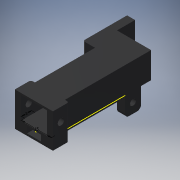
# Autodesk Inventor part: motoruchyt
Saved by Autodesk Inventor 2016 (Build 200138000, 138)
## iProperties
Created: 2015-05-23
Part Number: motoruchyt
Material: ABS Plastic
Document SubType Name: Modeling
Designer: Jufo
Density: 1 g/cm^3
Appearance: Smooth - White
Author: Jufo
Autodesk Inventor part; units mm, degrees
ref_plane "YZ Plane" through (0, 0, 0) normal (1, 0, 0) x (0, 1, 0)
ref_plane "XZ Plane" through (0, 0, 0) normal (0, 1, 0) x (-1, 0, 0)
ref_plane "XY Plane" through (0, 0, 0) normal (0, 0, 1) x (1, 0, 0)
sketch "Sketch1" plane through (0, 0, 0) normal (0, 1, 0) x (-1, 0, 0)
  line L0 (0, 6.5) -> (-5.5, 6.5)
  line L1 (-5.5, 6.5) -> (-5.5, -4.5)
  line L2 (-5.5, -4.5) -> (7.5, -4.5)
  line L3 (7.5, -4.5) -> (7.5, 6.5)
  line L4 (7.5, 6.5) -> (0, 6.5)
  line L5 (8.5, 7.5) -> (8.5, -5.5)
  line L6 (8.5, -5.5) -> (-6.5, -5.5)
  line L7 (-6.5, -5.5) -> (-6.5, 7.5)
  line L8 (-6.5, 7.5) -> (8.5, 7.5)
  point P0 (0, 0)
  dimension "d2" = 11
  dimension "d3" = 13
  dimension "d6" = 13
  dimension "d7" = 15
  dimension "d47" = 1
  dimension "d48" = 1
  constraints: 18 end point, 5 perpendicular, 1 collinear, 1 parallel
  measures "d2" distance of L0.end L1.end
  measures "d3" distance of L1.end L2.end
  measures "d6" distance of L5.start L5.end
  measures "d7" distance of L5.end L6.end
  measures "d47" distance between parallel lines of L8 L0
  measures "d48" distance between parallel lines of L1 L7
extrude "Extrusion1" add sketch "Sketch1" along normal blind 50
sketch "Sketch2" plane through (0, 50, 0) normal (0, 1, 0) x (1, 0, 0)
  line L0 (-8.5, 5.5) -> (-8.5, -7.5) projected
  line L1 (-8.5, -7.5) -> (6.5, -7.5) projected
  line L2 (6.5, -7.5) -> (6.5, 5.5) projected
  line L3 (6.5, 5.5) -> (-8.5, 5.5) projected
  circle A0 centre (0, 0) radius 2.5
  circle A1 centre (-4, 0) radius 0.75
  circle A2 centre (4, 0) radius 0.75
  dimension "d10" = 5
  dimension "d14" = 1.5
  constraints: 3 centre point, 1 coincident
  measures "d10" diameter of A0
  measures "d14" diameter of A1
extrude "Extrusion2" add sketch "Sketch2" along normal blind 1
sketch "Sketch3" plane through (6.5, 0, 7.5) normal (1, 0, 0) x (0, 0, -1)
  line L0 (0, 51) -> (13, 51) projected
  line L1 (0, 0) -> (0, 51) projected
  line L2 (6.5, 51) -> (6.5, 4)
  circle A0 centre (6.5, 4) radius 1.6
  point P0 (7.5, 0)
  dimension "d17" = 47
  dimension "d18" = 3.2
  constraints: 2 end point, 1 centre point, 1 coincident, 1 midpoint, 1 parallel
  measures "d17" distance of L2.start L2.end
  measures "d18" diameter of A0
extrude "Extrusion3" cut sketch "Sketch3" against normal blind 50
sketch "Sketch7" plane through (6.5, 0, -5.5) normal (0, 0, -1) x (-1, 0, 0)
  line L0 (0, 43) -> (0, 46)
  line L1 (0, 46) -> (4, 46)
  line L2 (4, 46) -> (4, 38)
  line L3 (4, 38) -> (0, 38)
  line L4 (0, 38) -> (0, 43)
  line L5 (11, 46) -> (11, 38)
  line L6 (11, 38) -> (15, 38)
  line L7 (15, 38) -> (15, 46)
  line L8 (15, 46) -> (11, 46)
  line L9 (0, 0) -> (0, 51) projected
  line L10 (0, 51) -> (15, 51) projected
  point P0 (6.5, 0)
  dimension "d33" = 3
  dimension "d34" = 8
  dimension "d35" = 7
  dimension "d36" = 4
  dimension "d37" = 4
  dimension "d38" = 8
  dimension "d55" = 0
  dimension "d92" = 7
  dimension "d93" = 5
  constraints: 18 end point, 4 perpendicular, 1 collinear, 1 parallel, 1 point on line
  measures "d33" distance of L0.start L0.end
  measures "d34" distance of L1.end L2.end
  measures "d35" distance of L1.end L5.start
  measures "d36" distance of L0.end L1.end
  measures "d37" distance of L5.end L6.end
  measures "d38" distance of L5.start L5.end
  measures "d55" distance between parallel lines of L9 L4
  measures "d92" distance of L5.end L2.end
  measures "d93" distance between parallel lines of L10 L1
extrude "Extrusion7" add sketch "Sketch7" along normal blind 10
sketch "Sketch9" plane through (0, 51, 0) normal (0, 1, 0) x (1, 0, 0)
  circle A0 centre (0, 0) radius 2.5 projected
  circle A1 centre (4, 0) radius 0.75 projected
  circle A2 centre (-4, 0) radius 0.75 projected
  circle A3 centre (-4, 0) radius 0.75
  circle A4 centre (4, 0) radius 0.75
  circle A5 centre (0, 0) radius 2.5
  constraints: 3 centre point, 3 coincident, 3 concentric
extrude "Extrusion9" add sketch "Sketch9" against normal blind 1
sketch "Sketch11" plane through (0, 51, 0) normal (0, 1, 0) x (1, 0, 0)
  line L0 (2.5, 5.5) -> (-4.5, 5.5) projected
  line L1 (6.5, 5.5) -> (-1, 5.5)
  line L2 (-1, 5.5) -> (-1, -1)
  circle A0 centre (-1, -1) radius 2.5
  point P0 (-17.5, 5.5)
  point P1 (0, 0)
  point P2 (-18.5, 5.5)
  point P3 (-8.5, 5.5)
  dimension "d51" = 7.5
  dimension "d52" = 5
  constraints: 4 end point, 1 centre point, 1 coincident, 1 midpoint, 1 perpendicular
  measures "d51" distance of L1.start L1.end
  measures "d52" diameter of A0
extrude "Extrusion10" cut sketch "Sketch11" against normal blind 1
sketch "Sketch12" plane through (6.5, 0, 7.5) normal (1, 0, 0) x (0, 0, -1)
  circle A0 centre (18.05, 42) radius 1.5
  line L0 (13, 38) -> (23, 38) projected
  line L1 (13, 46) -> (23, 46) projected
  point P0 (7.5, 0)
  dimension "d56" = 3
  dimension "d144" = 4
  dimension "d145" = 4
  constraints: 1 centre point
  measures "d56" diameter of A0
  measures "d144" distance from line of L0 A0.centre
  measures "d145" distance from line of A0.centre L1
extrude "Extrusion11" cut sketch "Sketch12" against normal blind 15
sketch "Sketch16" plane through (-8.5, 39, -13.5) normal (-1, 0, 0) x (0, 0, 1)
  line L0 (21, -39) -> (8, -39) projected
  circle A0 centre (14.5, -35) radius 1.6 projected
  line L1 (8, -39) -> (8, -1) projected
  line L2 (21, -39) -> (21, 12) projected
  line L3 (8, -31) -> (21, -31)
  dimension "d147" = 8
  constraints: 2 end point, 2 point on line, 1 perpendicular
  measures "d147" distance between parallel lines of L3 L0
extrude "Extrusion15" add sketch "Sketch16" along normal blind 2
sketch "Sketch17" plane through (6.5, 0, 7.5) normal (1, 0, 0) x (0, 0, -1)
  circle A0 centre (6.5, 4) radius 1.6 projected
  line L0 (0, 0) -> (0, 51) projected
  line L1 (13, 0) -> (0, 0) projected
  line L2 (13, 0) -> (13, 38) projected
  line L3 (13, 46) -> (23, 46) projected
  line L4 (6.5, 0) -> (6.5, 8)
  line L5 (0, 21) -> (13, 21)
  line L6 (0, 0) -> (0, 51) projected
  line L7 (0, 8) -> (13, 8)
  point P0 (7.5, 0)
  dimension "d78" = 8
  constraints: 6 end point, 4 point on line, 3 perpendicular, 1 midpoint
  measures "d78" distance of L4.start L4.end
fillet "Fillet11" radius 2 4 edges at (4.5, 46, -15.5) (4.5, 38, -15.5) (-6.5, 46, -15.5) (-6.5, 38, -15.5)
extrude "Extrusion18" add sketch "Sketch17" along normal blind 2 contours A0 L4 L7 L2 L1 | A0 L4 L1 L0 L7
sketch "Sketch21" plane through (-8.5, 8, 7.5) normal (-1, 0, 0) x (0, 0, 1)
  line L0 (-13, 52) -> (-13, 30)
  line L1 (0, 52) -> (0, 30)
  line L2 (0, 0) -> (0, 43) projected
  line L3 (-13, 38) -> (-13, 30) projected
  line L4 (-13, 30) -> (0, 30)
  line L5 (-13, 43) -> (0, 43) projected
  line L6 (-13, 52) -> (0, 52)
  constraints: 8 end point, 2 perpendicular, 1 horizontal, 1 point on line
extrude "Extrusion19" add sketch "Sketch21" along normal blind 6
sketch "Sketch31" plane through (0, 51, 0) normal (0, 1, 0) x (1, 0, 0)
  circle A0 centre (-1, -1) radius 2.5 projected
  line L0 (-1, -1) -> (3.45, -1)
  line L1 (5.5, -6.5) -> (5.5, 4.5) projected
  circle A1 centre (3.45, -1) radius 0.7
  line L2 (-1, -1) -> (-5.45, -1)
  circle A2 centre (-5.45, -1) radius 0.7
  point P0 (0, 0)
  dimension "d150" = 4.45
  dimension "d151" = 1.4
  dimension "d153" = 4.45
  dimension "d154" = 1.4
  dimension "d253" = 10.3
  constraints: 4 end point, 2 centre point, 2 coincident, 1 horizontal, 1 perpendicular
  measures "d150" distance of L0.start L0.end
  measures "d151" diameter of A1
  measures "d153" distance of L0.start L2.end
  measures "d154" diameter of A2
extrude "Extrusion28" cut sketch "Sketch31" against normal blind 2 contours A1 | A2
sketch "Sketch32" plane through (-14.5, 8, 7.5) normal (-1, 0, 0) x (0, 0, 1)
  line L0 (0, 30) -> (0, 52) projected
  line L1 (-13, 30) -> (0, 30) projected
  line L2 (-9.5, 50) -> (-3.5, 50)
  line L3 (-3.5, 50) -> (-3.5, 40)
  line L4 (-3.5, 40) -> (-9.5, 40)
  line L5 (-9.5, 40) -> (-9.5, 50)
  line L6 (-13, 52) -> (-13, 30) projected
  point P0 (-7.5, -8)
  dimension "d160" = 10
  dimension "d162" = 3.5
  dimension "d235" = 6
  dimension "d236" = 3.5
  constraints: 8 end point, 2 parallel, 1 horizontal, 1 perpendicular
  measures "d160" distance of L4.end L2.start
  measures "d162" distance between parallel lines of L0 L3
  measures "d235" distance of L2.start L2.end
  measures "d236" distance between parallel lines of L6 L5
extrude "Extrusion29" cut sketch "Sketch32" against normal blind 3
sketch "Sketch39" plane through (6.5, 46, -5.5) normal (0, 0, -1) x (-1, 0, 0)
  line L0 (4, 0) -> (4, -8) projected
  line L1 (-2, -46) -> (-2, -38) projected
  line L2 (-2, -46) -> (-2, -38)
  line L3 (0, -38) -> (-2, -38) projected
  line L4 (-2, -38) -> (0, -38)
  line L5 (0, -38) -> (0, -8)
  line L6 (0, -38) -> (0, -8) projected
  line L7 (0, -8) -> (4, -8)
  line L8 (15, -8) -> (11, -8) projected
  line L9 (11, -8) -> (15, -8)
  line L10 (15, -8) -> (15, -38)
  line L11 (15, -38) -> (17, -38) projected
  line L12 (15, -38) -> (17, -38)
  line L13 (17, -38) -> (17, -46) projected
  line L14 (17, -38) -> (17, -46)
  line L15 (17, -46) -> (-2, -46)
  line L16 (11, -8) -> (11, -46)
  line L17 (14, -46) -> (1, -46) projected
  line L18 (3, -8) -> (4, -8)
  line L19 (11, -8) -> (12, -8)
  line L20 (11, -8) -> (15, -8) projected
  line L21 (12, -8) -> (12, -46)
  line L22 (11, -46) -> (12, -46)
  line L23 (3, -8) -> (4, -8)
  line L24 (4, -8) -> (0, -8) projected
  line L25 (4, -8) -> (3, -8)
  line L26 (3, -8) -> (3, -46)
  line L27 (3, -46) -> (4, -46)
  line L28 (4, -46) -> (4, -8)
  line L29 (15, -38) -> (15, -8) projected
  line L30 (12, -8) -> (15, -8)
  line L31 (15, -8) -> (15, -13)
  line L32 (15, -13) -> (12, -13)
  line L33 (12, -13) -> (12, -8)
  line L34 (4, -8) -> (11, -8)
  line L35 (4, -9) -> (11, -9)
  line L36 (4, -9) -> (4, -12)
  line L37 (4, -9) -> (7, -9)
  arc A0 (7, -9) -> (4, -12) centre (7, -12) ccw
  line L38 (4, -12) -> (4, -46)
  line L39 (7, -9) -> (11, -9)
  line L40 (12, -38) -> (15, -38)
  line L41 (12, -39) -> (16, -39)
  line L42 (16, -39) -> (16, -45)
  line L43 (16, -45) -> (12, -45)
  line L44 (3, -45) -> (-1.4112, -45)
  line L45 (-1.4112, -45) -> (-1.4112, -39)
  line L46 (-1.4112, -39) -> (3, -39)
  line L47 (0, -38) -> (3, -38)
  line L48 (-2, -46) -> (17, -46) projected
  line L49 (3, -46) -> (-2, -46)
  line L50 (-2, -38) -> (-2, -46) projected
  line L51 (-2, -46) -> (-2, -38)
  line L52 (-2, -38) -> (3, -38)
  line L53 (11, -46) -> (17, -46)
  line L54 (17, -46) -> (17, -38) projected
  line L55 (17, -46) -> (17, -38)
  line L56 (17, -38) -> (12, -38)
  point P0 (6.5, -46)
  dimension "d218" = 1
  dimension "d230" = 5
  dimension "d234" = 1
  dimension "d242" = 3
  dimension "d243" = 3
  dimension "d255" = 1
  dimension "d256" = 1
  dimension "d257" = 1
  constraints: 86 end point, 17 point on line, 12 collinear, 12 perpendicular, 5 parallel, 4 horizontal, 2 point on circle, 1 centre point, 1 tangent, 1 vertical
  measures "d218" distance of L8.end L19.end
  measures "d230" distance of L30.end L31.end
  measures "d234" distance between parallel lines of L34 L35
  measures "d242" distance of L35.start L36.end
  measures "d243" distance of L35.start L37.end
  measures "d255" distance between parallel lines of L17 L43
  measures "d256" distance between parallel lines of L14 L42
  measures "d257" distance between parallel lines of L40 L41
extrude "Extrusion35" add sketch "Sketch39" along normal blind 3 contours L1 L3 L47 L26 L46 L45 L44 L15 | L26 L7 L28 L15 | L16 L8 L21 L15 | L28 L35 A0 | L34 L16 L35 L28 | L21 L43 L42 L41 L40 L11 L13 L15 | L8 L10 L32 L21
sketch "Sketch40" plane through (6.5, 46, -8.5) normal (0, 0, -1) x (-1, 0, 0)
  line L0 (15, -13) -> (12, -13) projected
  line L1 (12, -8) -> (15, -8)
  line L2 (15, -8) -> (15, -13)
  line L3 (15, -13) -> (12, -13)
  line L4 (0, -38) -> (-2, -38) projected
  line L5 (17, -46) -> (-2, -46)
  line L6 (-2, -46) -> (-2, -38)
  line L7 (-2, -38) -> (17, -38)
  line L8 (17, -38) -> (17, -46)
  line L9 (3, -38) -> (3, -8) projected
  line L10 (11, -38) -> (3, -38)
  line L11 (3, -38) -> (3, -8)
  line L12 (3, -8) -> (11, -8)
  line L13 (15, -13) -> (11, -13)
  line L14 (11, -13) -> (11, -8)
  line L15 (11, -8) -> (15, -8)
  line L16 (15, -8) -> (15, -13)
  line L17 (12, -38) -> (12, -13) projected
  line L18 (12, -38) -> (3, -38)
  line L19 (3, -38) -> (3, -13)
  line L20 (3, -13) -> (12, -13)
  line L21 (12, -13) -> (12, -38)
  point P0 (6.5, -46)
  point P1 (15, -38)
  constraints: 36 end point, 8 parallel, 5 horizontal, 5 perpendicular, 1 point on line
extrude "Extrusion36" add sketch "Sketch40" along normal blind 1
fillet "Fillet20" radius 1 2 edges at (-10.5, 8, -1) (8.5, 8, -1)
sketch "Sketch42" plane through (-8.5, 8, 7.5) normal (-1, 0, 0) x (0, 0, 1)
  circle A0 centre (-15, 27.3866) radius 1.5
  line L0 (-16.5, 25.8866) -> (-13.5, 25.8866)
  line L1 (-13.5, 25.8866) -> (-13.5, 28.8866)
  line L2 (-13.5, 28.8866) -> (-16.5, 28.8866)
  line L3 (-16.5, 28.8866) -> (-16.5, 25.8866)
  point P0 (-7.5, -8)
  dimension "d231" = 3
  constraints: 8 end point, 2 parallel, 1 centre point, 1 horizontal, 1 perpendicular
  measures "d231" diameter of A0
extrude "Extrusion38" cut sketch "Sketch42" against normal blind 5
sketch "Sketch43" plane through (-14.5, 48, 4) normal (0, 1, 0) x (1, 0, 0)
  circle A0 centre (2, 3) radius 1.5
  line L0 (4, 9.5) -> (4, -3.5) projected
  line L1 (3.5, 4.5) -> (0.5, 4.5)
  line L2 (0.5, 4.5) -> (0.5, 1.5)
  line L3 (0.5, 1.5) -> (3.5, 1.5)
  line L4 (3.5, 1.5) -> (3.5, 4.5)
  point P0 (14.5, 4)
  dimension "d237" = 3
  dimension "d238" = 2
  constraints: 8 end point, 2 parallel, 1 centre point, 1 horizontal, 1 perpendicular
  measures "d237" diameter of A0
  measures "d238" distance from line of L0 A0.centre
extrude "Extrusion39" cut sketch "Sketch43" against normal blind 15
fillet "Fillet21" radius 1 1 edges at (-14.5, 38, 1)
sketch "Sketch44" plane through (-8.5, 8, 7.5) normal (1, 0, 0) x (0, 0, -1)
  line L0 (13, 38) -> (13, 43) projected
  line L1 (0, 31) -> (0, 52) projected
  line L2 (13, 43) -> (0, 43)
  line L3 (0, 43) -> (0, 52)
  line L4 (0, 52) -> (13, 52)
  line L5 (13, 52) -> (13, 43)
  point P0 (7.5, -8)
  constraints: 8 end point, 2 parallel, 1 horizontal, 1 perpendicular
extrude "Extrusion40" cut sketch "Sketch44" against normal blind 2
fillet "Fillet24" radius 3 1 edges at (-11.5, 48, 1)
sketch "Sketch46" plane through (-7.5, 0, -4.5) normal (0, 0, 1) x (1, 0, 0)
  line L0 (15.4112, 1) -> (11, 1) projected
  line L1 (2, 7) -> (-2, 7) projected
  line L2 (15, 1) -> (-2, 1)
  line L3 (-2, 1) -> (-2, 7)
  line L4 (-2, 7) -> (15, 7)
  line L5 (15, 7) -> (15, 1)
  point P0 (7.5, 0)
  constraints: 8 end point, 2 parallel, 1 horizontal, 1 perpendicular, 1 point on line
extrude "Extrusion41" cut sketch "Sketch46" against normal blind 1
fillet "Fillet25" radius 3 1 edges at (-10.5, 60, 1)
body "Solid1"
